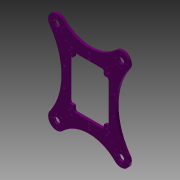
# Autodesk Inventor part: ATAS4baru
Saved by Autodesk Inventor 2015 (Build 190159000, 159)
## iProperties
Created: 2015-01-15
Part Number: ATAS4baru
Material: Generic
Document SubType Name: Modeling
Designer: Rafi Kurnia Putra
Density: 1 g/cm^3
Appearance: Smooth - Purple
Author: Rafi Kurnia Putra
Autodesk Inventor part; units mm, degrees
ref_plane "YZ Plane" through (0, 0, 0) normal (1, 0, 0) x (0, 1, 0)
ref_plane "XZ Plane" through (0, 0, 0) normal (0, 1, 0) x (-1, 0, 0)
ref_plane "XY Plane" through (0, 0, 0) normal (0, 0, 1) x (1, 0, 0)
sketch "Sketch1" plane through (0, 0, 0) normal (0, 1, 0) x (-1, 0, 0)
  arc A0 (39.6019, 0) -> (55.3297, -52.2069) centre (134.1138, 0) ccw
  circle A1 centre (28.625, -37.55) radius 1.75
  circle A2 centre (25.375, -42.175) radius 1.75
  arc A3 (37.9702, -69.5664) -> (0, -53.8386) centre (0, -107.5366) ccw
  circle A4 centre (46.65, -60.8866) radius 4.5
  arc A5 (37.9702, -69.5664) -> (55.3297, -52.2069) centre (46.65, -60.8866) ccw
  circle A6 centre (46.65, -60.8866) radius 4.5
  circle A7 centre (25.375, -42.175) radius 1.75
  circle A8 centre (28.625, -37.55) radius 1.75
  arc A9 (39.6019, 0) -> (55.3297, -52.2069) centre (134.1138, 0) ccw
  arc A10 (37.9702, -69.5664) -> (0, -53.8386) centre (0, -107.5366) ccw
  arc A11 (0, -42.175) -> (0, -38.675) centre (0, -40.425) ccw
  circle A12 centre (25.5, -34.24) radius 1.75
  arc A13 (37.9702, -69.5664) -> (55.3297, -52.2069) centre (46.65, -60.8866) ccw
  circle A14 centre (46.65, -69.3733) radius 1.25
  circle A15 centre (38.1633, -60.8866) radius 1.25
  circle A16 centre (55.1367, -60.8866) radius 1.25
  circle A17 centre (46.65, -52.3999) radius 1.25
  circle A18 centre (39.5789, -53.8156) radius 1.25
  circle A19 centre (33.215, -47.4516) radius 1.25
  line L0 (0, -37.55) -> (19.7877, -37.55)
  line L1 (21.7877, -35.55) -> (21.7877, -32)
  line L2 (28.625, -28) -> (28.625, 0)
  arc A20 (26.625, -30) -> (28.625, -28) centre (26.625, -28) ccw
  line L3 (23.7877, -30) -> (26.625, -30)
  arc A21 (23.7877, -30) -> (21.7877, -32) centre (23.7877, -32) ccw
  arc A22 (19.7877, -37.55) -> (21.7877, -35.55) centre (19.7877, -35.55) ccw
  arc A23 (0, -49.7631) -> (0, -46.2631) centre (0, -48.0131) ccw
  arc A24 (0, 38.675) -> (0, 42.175) centre (0, 40.425) ccw
  arc A25 (0, 53.8386) -> (37.9702, 69.5664) centre (0, 107.5366) ccw
  arc A26 (0, 53.8386) -> (37.9702, 69.5664) centre (0, 107.5366) ccw
  circle A27 centre (25.375, 42.175) radius 1.75
  circle A28 centre (25.375, 42.175) radius 1.75
  circle A29 centre (28.625, 37.55) radius 1.75
  circle A30 centre (28.625, 37.55) radius 1.75
  circle A31 centre (25.5, 34.24) radius 1.75
  arc A32 (55.3297, 52.2069) -> (39.6019, 0) centre (134.1138, 0) ccw
  arc A33 (55.3297, 52.2069) -> (39.6019, 0) centre (134.1138, 0) ccw
  circle A34 centre (46.65, 60.8866) radius 4.5
  arc A35 (55.3297, 52.2069) -> (37.9702, 69.5664) centre (46.65, 60.8866) ccw
  arc A36 (55.3297, 52.2069) -> (37.9702, 69.5664) centre (46.65, 60.8866) ccw
  circle A37 centre (46.65, 69.3733) radius 1.25
  circle A38 centre (38.1633, 60.8866) radius 1.25
  circle A39 centre (55.1367, 60.8866) radius 1.25
  circle A40 centre (46.65, 52.3999) radius 1.25
  circle A41 centre (39.5789, 53.8156) radius 1.25
  circle A42 centre (33.215, 47.4516) radius 1.25
  line L4 (0, 37.55) -> (19.7877, 37.55)
  line L5 (21.7877, 35.55) -> (21.7877, 32)
  line L6 (28.625, 28) -> (28.625, 0)
  arc A43 (28.625, 28) -> (26.625, 30) centre (26.625, 28) ccw
  line L7 (23.7877, 30) -> (26.625, 30)
  arc A44 (21.7877, 32) -> (23.7877, 30) centre (23.7877, 32) ccw
  arc A45 (21.7877, 35.55) -> (19.7877, 37.55) centre (19.7877, 35.55) ccw
  arc A46 (0, 46.2631) -> (0, 49.7631) centre (0, 48.0131) ccw
  arc A47 (0, -38.675) -> (0, -42.175) centre (0, -40.425) ccw
  arc A48 (0, -53.8386) -> (-37.9702, -69.5664) centre (0, -107.5366) ccw
  arc A49 (0, -53.8386) -> (-37.9702, -69.5664) centre (0, -107.5366) ccw
  circle A50 centre (-25.375, -42.175) radius 1.75
  circle A51 centre (-25.375, -42.175) radius 1.75
  circle A52 centre (-28.625, -37.55) radius 1.75
  circle A53 centre (-28.625, -37.55) radius 1.75
  circle A54 centre (-25.5, -34.24) radius 1.75
  arc A55 (-55.3297, -52.2069) -> (-39.6019, 0) centre (-134.1138, 0) ccw
  arc A56 (-55.3297, -52.2069) -> (-39.6019, 0) centre (-134.1138, 0) ccw
  circle A57 centre (-46.65, -60.8866) radius 4.5
  arc A58 (-55.3297, -52.2069) -> (-37.9702, -69.5664) centre (-46.65, -60.8866) ccw
  arc A59 (-55.3297, -52.2069) -> (-37.9702, -69.5664) centre (-46.65, -60.8866) ccw
  circle A60 centre (-46.65, -69.3733) radius 1.25
  circle A61 centre (-38.1633, -60.8866) radius 1.25
  circle A62 centre (-55.1367, -60.8866) radius 1.25
  circle A63 centre (-46.65, -52.3999) radius 1.25
  circle A64 centre (-39.5789, -53.8156) radius 1.25
  circle A65 centre (-33.215, -47.4516) radius 1.25
  line L8 (0, -37.55) -> (-19.7877, -37.55)
  line L9 (-21.7877, -35.55) -> (-21.7877, -32)
  line L10 (-28.625, -28) -> (-28.625, 0)
  arc A66 (-28.625, -28) -> (-26.625, -30) centre (-26.625, -28) ccw
  line L11 (-23.7877, -30) -> (-26.625, -30)
  arc A67 (-21.7877, -32) -> (-23.7877, -30) centre (-23.7877, -32) ccw
  arc A68 (-21.7877, -35.55) -> (-19.7877, -37.55) centre (-19.7877, -35.55) ccw
  arc A69 (0, -46.2631) -> (0, -49.7631) centre (0, -48.0131) ccw
  arc A70 (-19.7877, 37.55) -> (-21.7877, 35.55) centre (-19.7877, 35.55) ccw
  circle A71 centre (-28.625, 37.55) radius 1.75
  circle A72 centre (-28.625, 37.55) radius 1.75
  circle A73 centre (-33.215, 47.4516) radius 1.25
  circle A74 centre (-25.375, 42.175) radius 1.75
  circle A75 centre (-25.375, 42.175) radius 1.75
  arc A76 (-37.9702, 69.5664) -> (0, 53.8386) centre (0, 107.5366) ccw
  arc A77 (-37.9702, 69.5664) -> (0, 53.8386) centre (0, 107.5366) ccw
  arc A78 (0, 49.7631) -> (0, 46.2631) centre (0, 48.0131) ccw
  arc A79 (-39.6019, 0) -> (-55.3297, 52.2069) centre (-134.1138, 0) ccw
  arc A80 (-39.6019, 0) -> (-55.3297, 52.2069) centre (-134.1138, 0) ccw
  circle A81 centre (-38.1633, 60.8866) radius 1.25
  circle A82 centre (-39.5789, 53.8156) radius 1.25
  circle A83 centre (-46.65, 52.3999) radius 1.25
  circle A84 centre (-46.65, 69.3733) radius 1.25
  circle A85 centre (-46.65, 60.8866) radius 4.5
  arc A86 (-37.9702, 69.5664) -> (-55.3297, 52.2069) centre (-46.65, 60.8866) ccw
  arc A87 (-37.9702, 69.5664) -> (-55.3297, 52.2069) centre (-46.65, 60.8866) ccw
  circle A88 centre (-55.1367, 60.8866) radius 1.25
  circle A89 centre (-25.5, 34.24) radius 1.75
  line L12 (-21.7877, 35.55) -> (-21.7877, 32)
  line L13 (-23.7877, 30) -> (-26.625, 30)
  arc A90 (-26.625, 30) -> (-28.625, 28) centre (-26.625, 28) ccw
  arc A91 (0, 42.175) -> (0, 38.675) centre (0, 40.425) ccw
  line L14 (0, 37.55) -> (-19.7877, 37.55)
  line L15 (-28.625, 28) -> (-28.625, 0)
  arc A92 (-23.7877, 30) -> (-21.7877, 32) centre (-23.7877, 32) ccw
  arc A93 (-37.9702, 69.5664) -> (37.9702, 69.5664) centre (0, 107.5366) ccw
  arc A94 (37.9702, -69.5664) -> (-37.9702, -69.5664) centre (0, -107.5366) ccw
  arc A95 (55.3297, 52.2069) -> (55.3297, -52.2069) centre (134.1138, 0) ccw
  arc A96 (-55.3297, -52.2069) -> (-55.3297, 52.2069) centre (-134.1138, 0) ccw
  circle A97 centre (0, 40.425) radius 1.75
  circle A98 centre (0, -40.425) radius 1.75
  point P0 (4.2075, -54.5249)
  point P1 (4.2075, 54.5249)
  point P2 (-4.2075, -54.5249)
  point P3 (-4.2075, 54.5249)
  dimension "d2" = 4.625
  dimension "d3" = 3.5
  dimension "d4" = 3.5
  dimension "d10" = 3.5
  dimension "d15" = 2.5
  dimension "d16" = 2.5
  dimension "d17" = 2.5
  dimension "d18" = 2.5
  dimension "d20" = 10
  dimension "d21" = 2.5
  dimension "d22" = 2.5
  dimension "d23" = 9
  dimension "d30" = 2
  dimension "d31" = 2
  dimension "d42" = 9
  dimension "d43" = 9
  dimension "d44" = 9
  dimension "d45" = 9
  dimension "d46" = 2.5
  constraints: 108 point on circle, 99 centre point, 32 end point, 21 coincident, 7 tangent, 4 equal radius, 1 horizontal
  measures "d2" vertical distance of A2.centre A1.centre
  measures "d3" diameter of A2
  measures "d4" diameter of A1
  measures "d10" diameter of A12
  measures "d15" diameter of A14
  measures "d16" diameter of A15
  measures "d17" diameter of A16
  measures "d18" diameter of A17
  measures "d20" distance of point (39.579, -53.816) A4.centre
  measures "d21" diameter of A18
  measures "d22" diameter of A19
  measures "d23" distance of A19.centre A18.centre
  measures "d30" radius of A20
  measures "d31" radius of A21
  measures "d42" diameter of A57
  measures "d43" diameter of A85
  measures "d44" diameter of A4
  measures "d45" diameter of A34
  measures "d46" diameter of A62
extrude "Extrusion1" add sketch "Sketch1" along normal blind 3.5
sketch "Sketch2" plane through (0, 3.5, 0) normal (0, 1, 0) x (1, 0, 0)
  arc A0 (-55.3297, -52.2069) -> (-55.3297, 52.2069) centre (-134.1138, 0) ccw projected
  line L0 (-28.625, -28) -> (-28.625, 28) projected
  line L1 (-31.0417, 22.1386) -> (-31.0417, 21.017)
  spline S0 degree 2 poles (-31.0417, 21.017) (-31.0417, 19.8954) (-31.2164, 19.1001) (-31.9289, 18.5991) (-32.7057, 18.5991) knots 0 0 0 1 2 3 3 3
  spline S1 degree 2 poles (-32.7057, 18.5991) (-33.4183, 18.5991) (-33.9101, 18.953) (-33.9607, 19.4725) knots 0 0 0 1 2 2 2
  spline S2 degree 2 poles (-33.9607, 19.4725) (-34.0756, 19.0036) (-34.4663, 18.6772) (-34.7927, 18.5991) (-35.5328, 18.5991) knots 0 0 0 1 2 3 3 3
  line L2 (-35.5328, 18.5991) -> (-37.1417, 18.5991)
  line L3 (-37.1417, 18.5991) -> (-37.1417, 20.0747)
  line L4 (-37.1417, 20.0747) -> (-35.1145, 20.0747)
  spline S3 degree 2 poles (-35.1145, 20.0747) (-34.6272, 20.0747) (-34.3928, 20.2264) (-34.3928, 20.5527) knots 0 0 0 1 2 2 2
  line L5 (-34.3928, 20.5527) -> (-37.1417, 20.5527)
  line L6 (-37.1417, 20.5527) -> (-37.1417, 22.1386)
  line L7 (-37.1417, 22.1386) -> (-31.0417, 22.1386)
  line L8 (-32.0852, 20.5527) -> (-33.4412, 20.5527)
  spline S4 degree 2 poles (-33.4412, 20.5527) (-33.4412, 20.2861) (-33.2941, 20.0747) (-32.8896, 20.0747) knots 0 0 0 1 2 2 2
  line L9 (-32.8896, 20.0747) -> (-32.5541, 20.0747)
  spline S5 degree 2 poles (-32.5541, 20.0747) (-32.2645, 20.0747) (-32.0852, 20.2815) (-32.0852, 20.5527) knots 0 0 0 1 2 2 2
  spline S6 degree 2 poles (-34.6134, 11.6395) (-35.5328, 11.6395) (-36.2959, 11.7268) (-36.9302, 12.1819) (-37.2704, 12.9588) (-37.2704, 13.4736) knots 0 0 0 1 2 3 4 4 4
  spline S7 degree 2 poles (-37.2704, 13.4736) (-37.2704, 13.9655) (-36.9486, 14.7423) (-36.3097, 15.2158) (-35.5558, 15.3077) (-34.6134, 15.3077) knots 0 0 0 1 2 3 4 4 4
  line L10 (-34.6134, 15.3077) -> (-33.57, 15.3077)
  spline S8 degree 2 poles (-33.57, 15.3077) (-32.6506, 15.3077) (-31.8875, 15.2204) (-31.2531, 14.7653) (-30.913, 13.9885) (-30.913, 13.4736) knots 0 0 0 1 2 3 4 4 4
  spline S9 degree 2 poles (-30.913, 13.4736) (-30.913, 12.9817) (-31.2348, 12.2049) (-31.8737, 11.7314) (-32.6276, 11.6395) (-33.57, 11.6395) knots 0 0 0 1 2 3 4 4 4
  line L11 (-33.57, 11.6395) -> (-34.6134, 11.6395)
  spline S10 degree 2 poles (-32.6092, 13.2254) (-32.1863, 13.2254) (-31.9473, 13.3173) (-31.9473, 13.4644) knots 0 0 0 1 2 2 2
  spline S11 degree 2 poles (-31.9473, 13.4644) (-31.9473, 13.5885) (-32.1403, 13.7218) (-32.6092, 13.7218) knots 0 0 0 1 2 2 2
  line L12 (-32.6092, 13.7218) -> (-35.4547, 13.7218)
  spline S12 degree 2 poles (-35.4547, 13.7218) (-35.9879, 13.7218) (-36.2361, 13.6345) (-36.2361, 13.4782) knots 0 0 0 1 2 2 2
  spline S13 degree 2 poles (-36.2361, 13.4782) (-36.2361, 13.3173) (-35.9511, 13.2254) (-35.4133, 13.2254) knots 0 0 0 1 2 2 2
  line L13 (-35.4133, 13.2254) -> (-32.6092, 13.2254)
  line L14 (-31.0417, 8.3252) -> (-31.0417, 6.7438)
  spline S14 degree 2 poles (-31.0417, 6.7438) (-31.0417, 5.99) (-31.2761, 5.2177) (-31.9886, 4.7442) (-32.7793, 4.7442) knots 0 0 0 1 2 3 3 3
  spline S15 degree 2 poles (-32.7793, 4.7442) (-33.3125, 4.7442) (-33.7354, 5.0798) (-33.8458, 5.5762) knots 0 0 0 1 2 2 2
  spline S16 degree 2 poles (-33.8458, 5.5762) (-33.9745, 5.0246) (-34.5491, 4.6339) (-35.1467, 4.6339) knots 0 0 0 1 2 2 2
  line L15 (-35.1467, 4.6339) -> (-35.7075, 4.6339)
  spline S17 degree 2 poles (-35.7075, 4.6339) (-36.3281, 4.6339) (-36.921, 4.9143) (-37.1417, 5.5349) (-37.1417, 6.491) knots 0 0 0 1 2 3 3 3
  line L16 (-37.1417, 6.491) -> (-37.1417, 8.3252)
  line L17 (-37.1417, 8.3252) -> (-31.0417, 8.3252)
  line L18 (-34.3928, 6.7392) -> (-36.0982, 6.7392)
  spline S18 degree 2 poles (-36.0982, 6.7392) (-36.089, 6.4037) (-35.9005, 6.2198) (-35.5282, 6.2198) knots 0 0 0 1 2 2 2
  line L19 (-35.5282, 6.2198) -> (-34.9628, 6.2198)
  spline S19 degree 2 poles (-34.9628, 6.2198) (-34.5675, 6.2198) (-34.402, 6.3853) (-34.3928, 6.7392) knots 0 0 0 1 2 2 2
  line L20 (-32.0852, 6.7392) -> (-33.4412, 6.7392)
  spline S20 degree 2 poles (-33.4412, 6.7392) (-33.4366, 6.6381) (-33.4366, 6.583) knots 0 0 0 1 1 1
  spline S21 degree 2 poles (-33.4366, 6.583) (-33.4366, 6.3485) (-33.2068, 6.2198) (-32.6644, 6.2198) knots 0 0 0 1 2 2 2
  spline S22 degree 2 poles (-32.6644, 6.2198) (-32.3794, 6.2198) (-32.1495, 6.3255) (-32.0898, 6.4956) (-32.0852, 6.7392) knots 0 0 0 1 2 3 3 3
  line L21 (-31.0417, -2.2614) -> (-35.1191, -2.2614)
  spline S23 degree 2 poles (-35.1191, -2.2614) (-35.8132, -2.2614) (-36.374, -2.1694) (-36.967, -1.7281) (-37.2704, -1.0018) (-37.2704, -0.5054) knots 0 0 0 1 2 3 4 4 4
  spline S24 degree 2 poles (-37.2704, -0.5054) (-37.2704, 0.0417) (-36.9073, 0.8737) (-36.3281, 1.292) (-35.6845, 1.3655) (-34.6502, 1.3655) knots 0 0 0 1 2 3 4 4 4
  line L22 (-34.6502, 1.3655) -> (-31.0417, 1.3655)
  line L23 (-31.0417, 1.3655) -> (-31.0417, -0.2204)
  line L24 (-31.0417, -0.2204) -> (-35.6155, -0.2204)
  spline S25 degree 2 poles (-35.6155, -0.2204) (-36.0155, -0.2204) (-36.2361, -0.3077) (-36.2361, -0.4364) knots 0 0 0 1 2 2 2
  spline S26 degree 2 poles (-36.2361, -0.4364) (-36.2361, -0.5881) (-35.9925, -0.6754) (-35.5374, -0.6754) knots 0 0 0 1 2 2 2
  line L25 (-35.5374, -0.6754) -> (-31.0417, -0.6754)
  line L26 (-31.0417, -0.6754) -> (-31.0417, -2.2614)
  line L27 (-32.885, -8.9589) -> (-32.885, -7.4834)
  line L28 (-32.885, -7.4834) -> (-32.4345, -7.4834)
  spline S27 degree 2 poles (-32.4345, -7.4834) (-32.122, -7.4834) (-31.9473, -7.373) (-31.9473, -7.2397) knots 0 0 0 1 2 2 2
  spline S28 degree 2 poles (-31.9473, -7.2397) (-31.9473, -7.0972) (-32.1817, -6.9501) (-32.4161, -6.9501) knots 0 0 0 1 2 2 2
  spline S29 degree 2 poles (-32.4161, -6.9501) (-32.7195, -6.9501) (-32.8758, -7.0329) knots 0 0 0 1 1 1
  spline S30 degree 2 poles (-32.8758, -7.0329) (-33.0321, -7.1156) (-33.2482, -7.4834) knots 0 0 0 1 1 1
  spline S31 degree 2 poles (-33.2482, -7.4834) (-33.8779, -8.5406) (-34.2825, -8.8164) knots 0 0 0 1 1 1
  spline S32 degree 2 poles (-34.2825, -8.8164) (-34.687, -9.0923) (-35.5834, -9.0923) knots 0 0 0 1 1 1
  spline S33 degree 2 poles (-35.5834, -9.0923) (-36.2361, -9.0923) (-36.8521, -8.7889) (-37.2704, -7.9109) (-37.2704, -7.3317) knots 0 0 0 1 2 3 3 3
  spline S34 degree 2 poles (-37.2704, -7.3317) (-37.2704, -6.6973) (-36.7877, -5.7963) (-36.0431, -5.5159) (-35.3581, -5.5159) knots 0 0 0 1 2 3 3 3
  line L29 (-35.3581, -5.5159) -> (-34.9582, -5.5159)
  line L30 (-34.9582, -5.5159) -> (-34.9582, -6.9915)
  line L31 (-34.9582, -6.9915) -> (-35.6983, -6.9915)
  spline S35 degree 2 poles (-35.6983, -6.9915) (-36.0385, -6.9915) (-36.2361, -7.1156) (-36.2361, -7.2719) knots 0 0 0 1 2 2 2
  spline S36 degree 2 poles (-36.2361, -7.2719) (-36.2361, -7.4328) (-35.9879, -7.5845) (-35.7443, -7.5845) knots 0 0 0 1 2 2 2
  spline S37 degree 2 poles (-35.7443, -7.5845) (-35.2064, -7.5845) (-35.0409, -7.4374) knots 0 0 0 1 1 1
  spline S38 degree 2 poles (-35.0409, -7.4374) (-34.8755, -7.2857) (-34.4847, -6.6927) knots 0 0 0 1 1 1
  spline S39 degree 2 poles (-34.4847, -6.6927) (-34.094, -6.1043) (-33.74, -5.7182) (-33.1149, -5.4654) (-32.6276, -5.4654) knots 0 0 0 1 2 3 3 3
  spline S40 degree 2 poles (-32.6276, -5.4654) (-31.9243, -5.4654) (-31.2761, -5.8239) (-30.913, -6.6238) (-30.913, -7.1892) knots 0 0 0 1 2 3 3 3
  spline S41 degree 2 poles (-30.913, -7.1892) (-30.913, -7.8051) (-31.3129, -8.6785) (-31.9197, -8.9589) (-32.646, -8.9589) knots 0 0 0 1 2 3 3 3
  line L32 (-32.646, -8.9589) -> (-32.885, -8.9589)
  line L33 (-31.0417, -15.5048) -> (-32.2645, -15.5048)
  line L34 (-32.2645, -15.5048) -> (-32.2645, -14.5625)
  line L35 (-32.2645, -14.5625) -> (-37.1417, -14.5625)
  line L36 (-37.1417, -14.5625) -> (-37.1417, -12.9766)
  line L37 (-37.1417, -12.9766) -> (-32.2645, -12.9766)
  line L38 (-32.2645, -12.9766) -> (-32.2645, -12.0388)
  line L39 (-32.2645, -12.0388) -> (-31.0417, -12.0388)
  line L40 (-31.0417, -12.0388) -> (-31.0417, -15.5048)
  line L41 (-31.0417, -21.329) -> (-37.1417, -22.2392)
  line L42 (-37.1417, -22.2392) -> (-37.1417, -20.6119)
  line L43 (-37.1417, -20.6119) -> (-36.0431, -20.5292)
  line L44 (-36.0431, -20.5292) -> (-36.0431, -19.9638)
  line L45 (-36.0431, -19.9638) -> (-37.1417, -19.8718)
  line L46 (-37.1417, -19.8718) -> (-37.1417, -18.2262)
  line L47 (-37.1417, -18.2262) -> (-31.0417, -19.0306)
  line L48 (-31.0417, -19.0306) -> (-31.0417, -21.329)
  spline S42 degree 2 poles (-34.9628, -20.4878) (-33.9285, -20.3729) (-32.4024, -20.2488) knots 0 0 0 1 1 1
  spline S43 degree 2 poles (-32.4024, -20.2488) (-34.1538, -20.0097) (-34.9628, -19.9454) knots 0 0 0 1 1 1
  line L49 (-34.9628, -19.9454) -> (-34.9628, -20.4878)
  point P0 (0, 0)
  point P1 (-34.6353, -1.304)
  point P2 (-28.625, 0)
  point P3 (-34.0917, 0.0853)
  constraints: 1 midpoint, 2 other
extrude "Extrusion2" cut sketch "Sketch2" against normal blind 2.5
sketch "Sketch3" plane through (0, 3.5, 0) normal (0, 1, 0) x (1, 0, 0)
  circle A0 centre (-35.7085, 13.8987) radius 1.75
  circle A1 centre (35.7085, 13.8987) radius 1.75
  circle A2 centre (-35.7085, -13.8987) radius 1.75
  circle A3 centre (35.7085, -13.8987) radius 1.75
  constraints: 4 centre point, 1 coincident
extrude "Extrusion3" cut sketch "Sketch3" against normal through all
sketch "Sketch4" plane through (0, 0, 0) normal (0, -1, 0) x (1, 0, 0)
  circle A0 centre (-25.5, 34.24) radius 1.75 projected
  circle A1 centre (-25.5, -34.24) radius 1.75 projected
  circle A2 centre (25.5, 34.24) radius 1.75 projected
  point P0 (0, 0)
  dimension "d52" = 68.48
  dimension "d53" = 51
  measures "d52" distance of A1.centre A0.centre
  measures "d53" distance of A2.centre A0.centre
body "Solid1"
